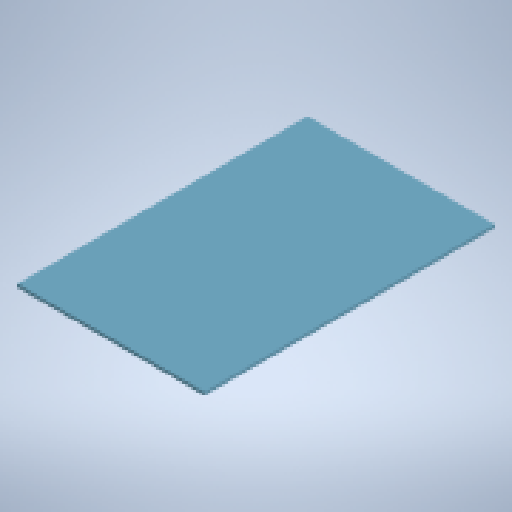
# Autodesk Inventor part: BaseCase
Saved by Autodesk Inventor 2024 (Build 280153000, 153)
## iProperties
Created: 2024-02-15
Part Number: BaseCase
Material: Generic
Document SubType Name: Modeling
Designer: fabiancastano
Density: 1 g/cm^3
Appearance: Default
Author: fabiancastano
Autodesk Inventor part; units mm, degrees
ref_plane "YZ Plane" through (0, 0, 0) normal (1, 0, 0) x (0, 1, 0)
ref_plane "XZ Plane" through (0, 0, 0) normal (0, 1, 0) x (-1, 0, 0)
ref_plane "XY Plane" through (0, 0, 0) normal (0, 0, 1) x (1, 0, 0)
sketch "Sketch1" plane through (0, 0, 0) normal (0, 1, 0) x (-1, 0, 0)
  line L0 (100, 155) -> (-100, 155)
  line L1 (-100, 155) -> (-100, -155)
  line L2 (-100, -155) -> (100, -155)
  line L3 (100, -155) -> (100, 155)
  point P0 (0, 0)
  point P1 (100, 0)
  point P2 (0, -155)
  dimension "d0" = 200
  dimension "d1" = 310
  constraints: 8 end point, 2 midpoint, 2 parallel, 1 horizontal, 1 horizontal alignment, 1 perpendicular, 1 vertical alignment
  measures "d0" distance of L2.end L1.end
  measures "d1" distance of L1.end L0.end
extrude "Extrusion1" add sketch "Sketch1" along normal blind 3.5
sketch "Sketch3" plane through (0, 3.5, 0) normal (0, 1, 0) x (1, 0, 0)
  line L0 (-80, 135) -> (-65, 135)
  line L1 (-65, 135) -> (-65, 120)
  line L2 (-65, 120) -> (-80, 120)
  line L3 (-80, 120) -> (-80, 135)
  line L4 (-31, 135) -> (-16, 135)
  line L5 (-16, 135) -> (-16, 120)
  line L6 (-16, 120) -> (-31, 120)
  line L7 (-31, 120) -> (-31, 135)
  line L8 (-80, 35.5) -> (-65, 35.5)
  line L9 (-65, 35.5) -> (-65, 20.5)
  line L10 (-65, 20.5) -> (-80, 20.5)
  line L11 (-80, 20.5) -> (-80, 35.5)
  line L12 (-31, 35.5) -> (-16, 35.5)
  line L13 (-16, 35.5) -> (-16, 20.5)
  line L14 (-16, 20.5) -> (-31, 20.5)
  line L15 (-31, 20.5) -> (-31, 35.5)
  line L16 (-80, -64) -> (-65, -64)
  line L17 (-65, -64) -> (-65, -79)
  line L18 (-65, -79) -> (-80, -79)
  line L19 (-80, -79) -> (-80, -64)
  line L20 (-31, -64) -> (-16, -64)
  line L21 (-16, -64) -> (-16, -79)
  line L22 (-16, -79) -> (-31, -79)
  line L23 (-31, -79) -> (-31, -64)
  line L24 (-100, 155) -> (-100, -155) projected
  line L25 (100, 155) -> (-100, 155) projected
  point P0 (0, 0)
  dimension "d4" = 15
  dimension "d5" = 15
  dimension "d8" = 49
  dimension "d11" = 99.5
  dimension "d14" = 20
  dimension "d15" = 20
  constraints: 48 end point, 2 collinear, 2 horizontal, 2 parallel, 1 perpendicular, 1 vertical, 38 other
  measures "d4" distance of L1.end L2.end
  measures "d5" distance of L0.end L1.end
  measures "d8" distance of L0.start L4.start
  measures "d11" distance of L0.start L8.start
  measures "d14" distance between parallel lines of L24 L3
  measures "d15" distance between parallel lines of L25 L0
extrude "Extrusion2" cut sketch "Sketch3" against normal blind 0.5
sketch "Sketch4" plane through (0, 3, 0) normal (0, 1, 0) x (1, 0, 0)
  line L0 (-65, 135) -> (-65, 120) projected
  line L1 (-65, 120) -> (-80, 120) projected
  line L2 (-65, 35.5) -> (-65, 20.5) projected
  line L3 (-31, 20.5) -> (-31, 35.5) projected
  line L4 (-80, -64) -> (-65, -64) projected
  line L5 (-31, -79) -> (-31, -64) projected
  point P0 (0, 0)
  point P1 (-69, 28)
  point P2 (-27, 28)
  point P3 (-69, -68)
  point P4 (-27, -68)
  point P5 (-69, 124)
  point P6 (-27, 124)
  point P7 (-65, 28)
  point P8 (-31, 28)
  dimension "d18" = 4
  dimension "d19" = 4
  dimension "d20" = 4
  dimension "d21" = 4
  constraints: 4 horizontal alignment, 4 vertical alignment, 2 midpoint
  measures "d18" distance from line of L0 point (-69, 124)
  measures "d19" distance from line of L1 point (-69, 124)
  measures "d20" distance from line of L4 point (-69, -68)
  measures "d21" distance from line of L5 point (-27, -68)
hole "Hole1" at (-69, 3, -28) at (-27, 3, -28) at (-69, 3, 68) at (-27, 3, 68) at (-69, 3, -124) at (-27, 3, -124) direction (0, -1, 0) diameter 3.5 end through all
body "Solid1"
